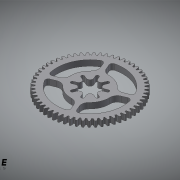
# Autodesk Inventor part: ギアm1z57
Saved by Autodesk Inventor 2020 (Build 240168000, 168)
## iProperties
Part Number: ギアm1z57
Material: 一般
Document SubType Name: Modeling
Designer: Kuroda Akito
Density: 1 g/cm^3
Appearance: 既定
Author: Kuroda Akito
Autodesk Inventor part; units mm, degrees
(part 1 of 3)
ref_plane "YZ Plane" through (0, 0, 0) normal (1, 0, 0) x (0, 1, 0)
ref_plane "XZ Plane" through (0, 0, 0) normal (0, 1, 0) x (-1, 0, 0)
ref_plane "XY Plane" through (0, 0, 0) normal (0, 0, 1) x (1, 0, 0)
sketch "スケッチ1" plane through (0, 0, 0) normal (0, 0, 1) x (1, 0, 0)
  arc A0 (149.035, 132.768) -> (148.9038, 132.247) centre (154.985, 130.9929) ccw
  arc A1 (149.2907, 133.5027) -> (149.035, 132.768) centre (157.2588, 130.3182) ccw
  arc A2 (149.7341, 134.4742) -> (149.2907, 133.5027) centre (159.5839, 129.3913) ccw
  arc A3 (145.977, 132.6583) -> (145.904, 132.1261) centre (152.0862, 131.5485) ccw
  arc A4 (146.1503, 133.4167) -> (145.977, 132.6583) centre (154.4205, 131.128) ccw
  arc A5 (146.4842, 134.431) -> (146.1503, 133.4167) centre (156.8334, 130.4626) ccw
  arc A6 (142.9497, 132.2129) -> (142.9356, 131.6758) centre (149.1439, 131.7819) ccw
  arc A7 (143.0385, 132.9857) -> (142.9497, 132.2129) centre (151.5102, 131.6208) ccw
  arc A8 (143.2588, 134.0307) -> (143.0385, 132.9857) centre (153.9817, 131.2248) ccw
  arc A9 (139.9898, 131.4372) -> (140.0349, 130.9018) centre (146.1937, 131.6901) ccw
  arc A10 (139.993, 132.2151) -> (139.9898, 131.4372) centre (148.5635, 131.7903) ccw
  arc A11 (140.097, 133.2779) -> (139.993, 132.2151) centre (151.0635, 131.6687) ccw
  arc A12 (137.1331, 130.3405) -> (137.2368, 129.8134) centre (143.2716, 131.2744) ccw
  arc A13 (137.0508, 131.1141) -> (137.1331, 130.3405) centre (145.6159, 131.6347) ccw
  arc A14 (137.0372, 132.1819) -> (137.0508, 131.1141) centre (148.1142, 131.7888) ccw
  arc A15 (134.4144, 128.9363) -> (134.5755, 128.4237) centre (140.4129, 130.5398) ccw
  arc A16 (134.2475, 129.6961) -> (134.4144, 128.9363) centre (142.7034, 131.1558) ccw
  arc A17 (134.1165, 130.7559) -> (134.2475, 129.6961) centre (145.1695, 131.5838) ccw
  arc A18 (131.8667, 127.2415) -> (132.0832, 126.7498) centre (137.6524, 129.4952) ccw
  arc A19 (131.6172, 127.9783) -> (131.8667, 127.2415) centre (139.8612, 130.3594) ccw
  arc A20 (131.3705, 129.0173) -> (131.6172, 127.9783) centre (142.2653, 131.0561) ccw
  arc A21 (129.5209, 125.2767) -> (129.7902, 124.8118) centre (135.0236, 128.1532) ccw
  arc A22 (129.1919, 125.9816) -> (129.5209, 125.2767) centre (137.1239, 129.2551) ccw
  arc A23 (128.8323, 126.9871) -> (129.1919, 125.9816) centre (139.4368, 130.2121) ccw
  arc A24 (127.4055, 123.0658) -> (127.7243, 122.6333) centre (132.5583, 126.5301) ccw
  arc A25 (127.0009, 123.7302) -> (127.4055, 123.0658) centre (134.5247, 127.8564) ccw
  arc A26 (126.5329, 124.69) -> (127.0009, 123.7302) centre (136.7182, 129.062) ccw
  arc A27 (125.5462, 120.6355) -> (125.9106, 120.2408) centre (130.2866, 124.6457) ccw
  arc A28 (125.0709, 121.2514) -> (125.5462, 120.6355) centre (132.0951, 126.1803) ccw
  arc A29 (124.5002, 122.154) -> (125.0709, 121.2514) centre (134.1427, 127.6199) ccw
  arc A30 (123.9655, 118.0155) -> (124.3711, 117.6632) centre (128.2359, 122.5229) ccw
  arc A31 (123.4253, 118.5754) -> (123.9655, 118.0155) centre (129.8647, 124.2471) ccw
  arc A32 (122.7588, 119.4097) -> (123.4253, 118.5754) centre (131.7415, 125.9032) ccw
  arc A33 (122.6825, 115.2375) -> (123.1245, 114.932) centre (126.4313, 120.1873) ccw
  arc A34 (122.0841, 115.7346) -> (122.6825, 115.2375) centre (127.8604, 122.0802) ccw
  arc A35 (121.3298, 116.4905) -> (122.0841, 115.7346) centre (129.5437, 123.9327) ccw
  arc A36 (121.713, 112.3353) -> (122.1859, 112.0802) centre (124.8945, 117.6674) ccw
  arc A37 (121.0636, 112.7635) -> (121.713, 112.3353) centre (126.1067, 119.7061) ccw
  arc A38 (120.2307, 113.4318) -> (121.0636, 112.7635) centre (127.576, 121.7325) ccw
  arc A39 (121.0687, 109.344) -> (121.5667, 109.1425) centre (123.6442, 114.9937) ccw
  arc A40 (120.376, 109.6981) -> (121.0687, 109.344) centre (124.6249, 117.1534) ccw
  arc A41 (119.4747, 110.2708) -> (120.376, 109.6981) centre (125.8623, 119.3291) ccw
  arc A42 (120.7573, 106.2999) -> (121.2745, 106.1544) centre (122.6957, 112.1987) ccw
  arc A43 (120.0299, 106.5757) -> (120.7573, 106.2999) centre (123.4328, 114.4531) ccw
  arc A44 (119.071, 107.0458) -> (120.0299, 106.5757) centre (124.4233, 116.7518) ccw
  arc A45 (120.7827, 103.2401) -> (121.3127, 103.1524) centre (122.0604, 109.3163) ccw
  arc A46 (120.0294, 103.4342) -> (120.7827, 103.2401) centre (122.545, 111.6382) ccw
  arc A47 (119.0246, 103.7959) -> (120.0294, 103.4342) centre (123.2767, 114.0318) ccw
  arc A48 (121.1445, 100.2017) -> (121.681, 100.1728) centre (121.746, 106.3816) ccw
  arc A49 (120.3744, 100.3117) -> (121.1445, 100.2017) centre (121.9723, 108.7426) ccw
  arc A50 (119.3359, 100.5607) -> (120.3744, 100.3117) centre (122.4362, 111.2023) ccw
  arc A51 (121.8384, 97.2214) -> (122.3748, 97.2518) centre (121.7564, 103.43) ccw
  arc A52 (121.0608, 97.2461) -> (121.8384, 97.2214) centre (121.7216, 105.8016) ccw
  arc A53 (120.0013, 97.3793) -> (121.0608, 97.2461) centre (121.9121, 108.2974) ccw
  arc A54 (122.8559, 94.3357) -> (123.3857, 94.4248) centre (122.0915, 100.4975) ccw
  arc A55 (122.0804, 94.2747) -> (122.8559, 94.3357) centre (121.7959, 102.8509) ccw
  arc A56 (121.0126, 94.2905) -> (122.0804, 94.2747) centre (121.7107, 105.3525) ccw
  arc A57 (124.1847, 91.5793) -> (124.7015, 91.7262) centre (122.7471, 97.6197) ccw
  arc A58 (123.4206, 91.4334) -> (124.1847, 91.5793) centre (122.1944, 99.9263) ccw
  arc A59 (122.3576, 91.3317) -> (123.4206, 91.4334) centre (121.8345, 102.4033) ccw
  arc A60 (125.8087, 88.9859) -> (126.3062, 89.1887) centre (123.7152, 94.8315) ccw
  arc A61 (125.0653, 88.7568) -> (125.8087, 88.9859) centre (122.9122, 97.0632) ccw
  arc A62 (124.0199, 88.5387) -> (125.0653, 88.7568) centre (122.282, 99.4856) ccw
  arc A63 (127.7081, 86.5869) -> (128.1802, 86.8432) centre (124.9843, 92.1667) ccw
  arc A64 (126.9944, 86.2773) -> (127.7081, 86.5869) centre (123.9406, 94.2966) ccw
  arc A65 (125.9793, 85.9456) -> (126.9944, 86.2773) centre (123.0478, 96.6349) ccw
  arc A66 (129.8599, 84.4113) -> (130.3009, 84.7181) centre (126.5388, 89.6576) ccw
  arc A67 (129.1845, 84.0252) -> (129.8599, 84.4113) centre (125.2672, 91.6598) ccw
  arc A68 (128.2121, 83.5838) -> (129.1845, 84.0252) centre (124.1225, 93.8857) ccw
  arc A69 (132.2379, 82.4857) -> (132.6426, 82.8391) centre (128.3599, 87.3348) ccw
  arc A70 (131.6092, 82.0276) -> (132.2379, 82.4857) centre (126.8757, 89.1849) ccw
  arc A71 (130.6912, 81.482) -> (131.6092, 82.0276) centre (125.4931, 91.2715) ccw
  arc A72 (134.8134, 80.8334) -> (135.1767, 81.2292) centre (130.4254, 85.2265) ccw
  arc A73 (134.2388, 80.3089) -> (134.8134, 80.8334) centre (128.7467, 86.9021) ccw
  arc A74 (133.3865, 79.6656) -> (134.2388, 80.3089) centre (127.143, 88.8238) ccw
  arc A75 (137.555, 79.4744) -> (137.8726, 79.9078) centre (132.7104, 83.3581) ccw
  arc A76 (137.0416, 78.8899) -> (137.555, 79.4744) centre (130.8575, 84.8389) ccw
  arc A77 (136.2652, 78.1567) -> (137.0416, 78.8899) centre (129.0521, 86.5726) ccw
  arc A78 (140.4294, 78.4253) -> (140.6974, 78.891) centre (135.187, 81.7525) ccw
  arc A79 (139.9835, 77.7879) -> (140.4294, 78.4253) centre (133.1825, 83.0204) ccw
  arc A80 (139.2925, 76.9737) -> (139.9835, 77.7879) centre (131.1973, 84.545) ccw
  arc A81 (143.4018, 77.6988) -> (143.617, 78.1911) centre (137.8252, 80.429) ccw
  arc A82 (143.0287, 77.0162) -> (143.4018, 77.6988) centre (135.6934, 81.4688) ccw
  arc A83 (142.4315, 76.1309) -> (143.0287, 77.0162) centre (133.5526, 82.7657) ccw
  arc A84 (146.4361, 77.3036) -> (146.5958, 77.8166) centre (140.593, 79.4039) ccw
  arc A85 (146.1404, 76.5841) -> (146.4361, 77.3036) centre (138.3598, 80.2028) ccw
  arc A86 (145.6441, 75.6386) -> (146.1404, 76.5841) centre (136.0892, 81.2563) ccw
  arc A87 (149.4955, 77.2447) -> (149.5978, 77.7721) centre (143.4568, 78.6894) ccw
  arc A88 (149.2807, 76.497) -> (149.4955, 77.2447) centre (141.1492, 79.2378) ccw
  arc A89 (148.8915, 75.5026) -> (149.2807, 76.497) centre (138.7766, 80.0351) ccw
  arc A90 (152.5428, 77.5227) -> (152.5864, 78.0581) centre (146.3818, 78.2943) ccw
  arc A91 (152.4115, 76.7559) -> (152.5428, 77.5227) centre (144.0279, 78.5855) ccw
  arc A92 (152.134, 75.7247) -> (152.4115, 76.7559) centre (141.5819, 79.117) ccw
  arc A93 (155.541, 78.1342) -> (155.5254, 78.6712) centre (149.3325, 78.2233) ccw
  arc A94 (155.4949, 77.3576) -> (155.541, 78.1342) centre (146.9608, 78.2538) ccw
  arc A95 (155.3325, 76.3021) -> (155.4949, 77.3576) centre (144.4713, 78.513) ccw
  arc A96 (158.4537, 79.0718) -> (158.3792, 79.6038) centre (152.2731, 78.4774) ccw
  arc A97 (158.4933, 78.2949) -> (158.4537, 79.0718) centre (149.9125, 78.2468) ccw
  arc A98 (158.448, 77.228) -> (158.4933, 78.2949) centre (147.4095, 78.2306) ccw
  arc A99 (161.2456, 80.3241) -> (161.113, 80.8448) centre (155.1679, 79.0535) ccw
  arc A100 (161.3704, 79.5563) -> (161.2456, 80.3241) centre (152.847, 78.5646) ccw
  arc A101 (161.4428, 78.4909) -> (161.3704, 79.5563) centre (150.361, 78.2731) ccw
  arc A102 (163.8828, 81.876) -> (163.6937, 82.3789) centre (157.9817, 79.9445) ccw
  arc A103 (164.0913, 81.1266) -> (163.8828, 81.876) centre (155.7287, 79.2032) ccw
  arc A104 (164.2805, 80.0756) -> (164.0913, 81.1266) centre (153.2899, 78.64) ccw
  arc A105 (166.3332, 83.7086) -> (166.09, 84.1876) centre (160.6805, 81.1396) ccw
  arc A106 (166.623, 82.9867) -> (166.3332, 83.7086) centre (158.5227, 80.155) ccw
  arc A107 (166.9266, 81.9628) -> (166.623, 82.9867) centre (156.1606, 79.3269) ccw
  arc A108 (168.5672, 85.7996) -> (168.2728, 86.249) centre (163.2314, 82.6244) ccw
  arc A109 (168.9346, 85.1139) -> (168.5672, 85.7996) centre (161.195, 81.4084) ccw
  arc A110 (169.349, 84.1297) -> (168.9346, 85.1139) centre (158.9383, 80.3255) ccw
  arc A111 (170.5576, 88.1237) -> (170.2155, 88.538) centre (165.6035, 84.3808) ccw
  arc A112 (170.9982, 87.4826) -> (170.5576, 88.1237) centre (163.7132, 82.9481) ccw
  arc A113 (171.5184, 86.55) -> (170.9982, 87.4826) centre (161.5894, 81.6236) ccw
  arc A114 (172.2803, 90.6527) -> (171.8947, 91.0268) centre (167.768, 86.3874) ccw
  arc A115 (172.7887, 90.0639) -> (172.2803, 90.6527) centre (166.0468, 84.7555) ccw
  arc A116 (173.4083, 89.1942) -> (172.7887, 90.0639) centre (164.0815, 83.2054) ccw
  arc A117 (173.7143, 93.3558) -> (173.2899, 93.6852) centre (169.6986, 88.62) ccw
  arc A118 (174.2844, 92.8265) -> (173.7143, 93.3558) centre (168.1673, 86.8087) ccw
  arc A119 (174.9959, 92.0302) -> (174.2844, 92.8265) centre (166.3846, 85.0518) ccw
  arc A120 (174.8422, 96.2002) -> (174.3841, 96.481) centre (171.3719, 91.0515) ccw
  arc A121 (175.4671, 95.7369) -> (174.8422, 96.2002) centre (170.0491, 89.0827) ccw
  arc A122 (176.2619, 95.0237) -> (175.4671, 95.7369) centre (168.4705, 87.1403) ccw
  arc A123 (175.6504, 99.1515) -> (175.1642, 99.3801) centre (172.7675, 93.6522) ccw
  arc A124 (176.3224, 98.7597) -> (175.6504, 99.1515) centre (171.6694, 91.5499) ccw
  arc A125 (177.1909, 98.1383) -> (176.3224, 98.7597) centre (170.314, 89.4456) ccw
  arc A126 (176.129, 102.1738) -> (175.6206, 102.3475) centre (173.8685, 96.3907) ccw
  arc A127 (176.8401, 101.8583) -> (176.129, 102.1738) centre (173.0084, 94.1803) ccw
  arc A128 (177.7716, 101.3362) -> (176.8401, 101.8583) centre (171.8927, 91.9397) ccw
  arc A129 (176.2722, 105.2303) -> (175.7478, 105.3471) centre (174.6617, 99.2337) ccw
  arc A130 (177.0137, 104.995) -> (176.2722, 105.2303) centre (174.0499, 96.9421) ccw
  arc A131 (177.997, 104.5785) -> (177.0137, 104.995) centre (173.1875, 94.5924) ccw
  arc A132 (176.0783, 108.2841) -> (175.5442, 108.3425) centre (175.1372, 102.1467) ccw
  arc A133 (176.8412, 108.1318) -> (176.0783, 108.2841) centre (174.7813, 99.8017) ccw
  arc A134 (177.8643, 107.826) -> (176.8412, 108.1318) centre (174.1826, 97.3714) ccw
  arc A135 (175.5496, 111.298) -> (175.0124, 111.2973) centre (175.2894, 105.0943) ccw
  arc A136 (176.3246, 111.2305) -> (175.5496, 111.298) centre (175.1936, 102.7244) ccw
  arc A137 (177.3752, 111.0392) -> (176.3246, 111.2305) centre (174.8659, 100.243) ccw
  arc A138 (174.6926, 114.2355) -> (174.1587, 114.1756) centre (175.1165, 108.0408) ccw
  arc A139 (175.4703, 114.2537) -> (174.6926, 114.2355) centre (175.2819, 105.6748) ccw
  arc A140 (176.5356, 114.179) -> (175.4703, 114.2537) centre (175.2292, 103.1723) ccw
  arc A141 (173.5177, 117.0608) -> (172.9936, 116.9426) centre (174.6204, 110.9504) ccw
  arc A142 (174.2887, 117.1645) -> (173.5177, 117.0608) centre (175.0451, 108.6169) ccw
  arc A143 (175.3557, 117.2075) -> (174.2887, 117.1645) centre (175.268, 106.1238) ccw
  arc A144 (172.0391, 119.7398) -> (171.5312, 119.5646) centre (173.8073, 113.7878) ccw
  arc A145 (172.794, 119.9276) -> (172.0391, 119.7398) centre (174.4861, 111.5151) ccw
  arc A146 (173.8498, 120.0877) -> (172.794, 119.9276) centre (174.9819, 109.0617) ccw
  arc A147 (170.2747, 122.2398) -> (169.7891, 122.0099) centre (172.687, 116.5184) ccw
  arc A148 (171.0044, 122.5095) -> (170.2747, 122.2398) centre (173.6117, 114.3343) ccw
  arc A149 (172.0361, 122.7848) -> (171.0044, 122.5095) centre (174.3744, 111.9503) ccw
  arc A150 (168.246, 124.5306) -> (167.7887, 124.2486) centre (171.273, 119.1093) ccw
  arc A151 (168.9416, 124.8789) -> (168.246, 124.5306) centre (172.4325, 117.0401) ccw
  arc A152 (169.9368, 125.2661) -> (168.9416, 124.8789) centre (173.4528, 114.7545) ccw
  arc A153 (165.9777, 126.5843) -> (165.5541, 126.2537) centre (169.5827, 121.5289) ccw
  arc A154 (166.6307, 127.007) -> (165.9777, 126.5843) centre (170.9627, 119.5998) ccw
  arc A155 (167.5773, 127.5013) -> (166.6307, 127.007) centre (172.2282, 117.4403) ccw
  arc A156 (163.4971, 128.3759) -> (163.1125, 128.0008) centre (167.6364, 123.7478) ccw
  arc A157 (164.0997, 128.868) -> (163.4971, 128.3759) centre (169.2203, 121.9823) ccw
  arc A158 (164.9862, 129.4634) -> (164.0997, 128.868) centre (170.7157, 119.9751) ccw
  arc A159 (160.8346, 129.8839) -> (160.4936, 129.4687) centre (165.4579, 125.7392) ccw
  arc A160 (161.3793, 130.4392) -> (160.8346, 129.8839) centre (167.2263, 124.1586) ccw
  arc A161 (162.1949, 131.1285) -> (161.3793, 130.4392) centre (168.9335, 122.3281) ccw
  arc A162 (158.0223, 131.0897) -> (157.729, 130.6396) centre (163.0734, 127.4788) ccw
  arc A163 (158.5026, 131.7016) -> (158.0223, 131.0897) centre (165.005, 126.1024) ccw
  arc A164 (159.2375, 132.4765) -> (158.5026, 131.7016) centre (166.9032, 124.4708) ccw
  arc A165 (155.0944, 131.9789) -> (154.8525, 131.4992) centre (160.5121, 128.9456) ccw
  arc A166 (155.5045, 132.6399) -> (155.0944, 131.9789) centre (162.5834, 127.79) ccw
  arc A167 (156.1497, 133.4909) -> (155.5045, 132.6399) centre (164.6496, 126.3771) ccw
  arc A168 (152.0865, 132.5406) -> (151.8988, 132.0372) centre (157.805, 130.1217) ccw
  arc A169 (152.4214, 133.2427) -> (152.0865, 132.5406) centre (159.9909, 129.201) ccw
  arc A170 (152.969, 134.1595) -> (152.4214, 133.2427) centre (162.1999, 128.024) ccw
  arc A171 (148.0962, 132.247) -> (147.965, 132.768) centre (142.015, 130.9929) ccw
  arc A172 (147.965, 132.768) -> (147.7093, 133.5027) centre (139.7412, 130.3182) ccw
  arc A173 (147.7093, 133.5027) -> (147.2659, 134.4742) centre (137.4161, 129.3913) ccw
  arc A174 (145.1012, 132.0372) -> (144.9135, 132.5406) centre (139.195, 130.1217) ccw
  arc A175 (144.9135, 132.5406) -> (144.5786, 133.2427) centre (137.0091, 129.201) ccw
  arc A176 (144.5786, 133.2427) -> (144.031, 134.1595) centre (134.8001, 128.024) ccw
  arc A177 (142.1475, 131.4992) -> (141.9056, 131.9789) centre (136.4879, 128.9456) ccw
  arc A178 (141.9056, 131.9789) -> (141.4955, 132.6399) centre (134.4166, 127.79) ccw
  arc A179 (141.4955, 132.6399) -> (140.8503, 133.4909) centre (132.3504, 126.3771) ccw
  arc A180 (139.271, 130.6396) -> (138.9777, 131.0897) centre (133.9266, 127.4788) ccw
  arc A181 (138.9777, 131.0897) -> (138.4974, 131.7016) centre (131.995, 126.1024) ccw
  arc A182 (138.4974, 131.7016) -> (137.7625, 132.4765) centre (130.0968, 124.4708) ccw
  arc A183 (136.5064, 129.4687) -> (136.1654, 129.8839) centre (131.5421, 125.7392) ccw
  arc A184 (136.1654, 129.8839) -> (135.6207, 130.4392) centre (129.7737, 124.1586) ccw
  arc A185 (135.6207, 130.4392) -> (134.8051, 131.1285) centre (128.0665, 122.3281) ccw
  arc A186 (133.8875, 128.0008) -> (133.5029, 128.3759) centre (129.3636, 123.7478) ccw
  arc A187 (133.5029, 128.3759) -> (132.9003, 128.868) centre (127.7797, 121.9823) ccw
  arc A188 (132.9003, 128.868) -> (132.0138, 129.4634) centre (126.2843, 119.9751) ccw
  arc A189 (131.4459, 126.2537) -> (131.0223, 126.5843) centre (127.4173, 121.5289) ccw
  arc A190 (131.0223, 126.5843) -> (130.3693, 127.007) centre (126.0373, 119.5998) ccw
  arc A191 (130.3693, 127.007) -> (129.4227, 127.5013) centre (124.7718, 117.4403) ccw
  arc A192 (129.2113, 124.2486) -> (128.754, 124.5306) centre (125.727, 119.1093) ccw
  arc A193 (128.754, 124.5306) -> (128.0584, 124.8789) centre (124.5675, 117.0401) ccw
  arc A194 (128.0584, 124.8789) -> (127.0632, 125.2661) centre (123.5472, 114.7545) ccw
  arc A195 (127.2109, 122.0099) -> (126.7253, 122.2398) centre (124.313, 116.5184) ccw
  arc A196 (126.7253, 122.2398) -> (125.9956, 122.5095) centre (123.3883, 114.3343) ccw
  arc A197 (125.9956, 122.5095) -> (124.9639, 122.7848) centre (122.6256, 111.9503) ccw
  arc A198 (125.4688, 119.5646) -> (124.9609, 119.7398) centre (123.1927, 113.7878) ccw
  arc A199 (124.9609, 119.7398) -> (124.206, 119.9276) centre (122.5139, 111.5151) ccw
  arc A200 (124.206, 119.9276) -> (123.1502, 120.0877) centre (122.0181, 109.0617) ccw
  arc A201 (124.0064, 116.9426) -> (123.4823, 117.0608) centre (122.3796, 110.9504) ccw
  arc A202 (123.4823, 117.0608) -> (122.7113, 117.1645) centre (121.9549, 108.6169) ccw
  arc A203 (122.7113, 117.1645) -> (121.6443, 117.2075) centre (121.732, 106.1238) ccw
  arc A204 (122.8413, 114.1756) -> (122.3074, 114.2355) centre (121.8835, 108.0408) ccw
  arc A205 (122.3074, 114.2355) -> (121.5297, 114.2537) centre (121.7181, 105.6748) ccw
  arc A206 (121.5297, 114.2537) -> (120.4644, 114.179) centre (121.7708, 103.1723) ccw
  arc A207 (121.9876, 111.2973) -> (121.4504, 111.298) centre (121.7106, 105.0943) ccw
  arc A208 (121.4504, 111.298) -> (120.6754, 111.2305) centre (121.8064, 102.7244) ccw
  arc A209 (120.6754, 111.2305) -> (119.6248, 111.0392) centre (122.1341, 100.243) ccw
  arc A210 (121.4558, 108.3425) -> (120.9217, 108.2841) centre (121.8628, 102.1467) ccw
  arc A211 (120.9217, 108.2841) -> (120.1588, 108.1318) centre (122.2187, 99.8017) ccw
  arc A212 (120.1588, 108.1318) -> (119.1357, 107.826) centre (122.8174, 97.3714) ccw
  arc A213 (121.2522, 105.3471) -> (120.7278, 105.2303) centre (122.3383, 99.2337) ccw
  arc A214 (120.7278, 105.2303) -> (119.9863, 104.995) centre (122.9501, 96.9421) ccw
  arc A215 (119.9863, 104.995) -> (119.003, 104.5785) centre (123.8125, 94.5924) ccw
  arc A216 (121.3794, 102.3475) -> (120.871, 102.1738) centre (123.1315, 96.3907) ccw
  arc A217 (120.871, 102.1738) -> (120.1599, 101.8583) centre (123.9916, 94.1803) ccw
  arc A218 (120.1599, 101.8583) -> (119.2284, 101.3362) centre (125.1073, 91.9397) ccw
  arc A219 (121.8358, 99.3801) -> (121.3496, 99.1515) centre (124.2325, 93.6522) ccw
  arc A220 (121.3496, 99.1515) -> (120.6776, 98.7597) centre (125.3306, 91.5499) ccw
  arc A221 (120.6776, 98.7597) -> (119.8091, 98.1383) centre (126.686, 89.4456) ccw
  arc A222 (122.6159, 96.481) -> (122.1578, 96.2002) centre (125.6281, 91.0515) ccw
  arc A223 (122.1578, 96.2002) -> (121.5329, 95.7369) centre (126.9509, 89.0827) ccw
  arc A224 (121.5329, 95.7369) -> (120.7381, 95.0237) centre (128.5295, 87.1403) ccw
  arc A225 (123.7101, 93.6852) -> (123.2857, 93.3558) centre (127.3014, 88.62) ccw
  arc A226 (123.2857, 93.3558) -> (122.7156, 92.8265) centre (128.8327, 86.8087) ccw
  arc A227 (122.7156, 92.8265) -> (122.0041, 92.0302) centre (130.6154, 85.0518) ccw
  arc A228 (125.1053, 91.0268) -> (124.7197, 90.6527) centre (129.232, 86.3874) ccw
  arc A229 (124.7197, 90.6527) -> (124.2113, 90.0639) centre (130.9532, 84.7555) ccw
  arc A230 (124.2113, 90.0639) -> (123.5917, 89.1942) centre (132.9185, 83.2054) ccw
  arc A231 (126.7845, 88.538) -> (126.4424, 88.1237) centre (131.3965, 84.3808) ccw
  arc A232 (126.4424, 88.1237) -> (126.0018, 87.4826) centre (133.2868, 82.9481) ccw
  arc A233 (126.0018, 87.4826) -> (125.4816, 86.55) centre (135.4106, 81.6236) ccw
  arc A234 (128.7272, 86.249) -> (128.4328, 85.7996) centre (133.7686, 82.6244) ccw
  arc A235 (128.4328, 85.7996) -> (128.0654, 85.1139) centre (135.805, 81.4084) ccw
  arc A236 (128.0654, 85.1139) -> (127.651, 84.1297) centre (138.0617, 80.3255) ccw
  arc A237 (130.91, 84.1876) -> (130.6668, 83.7086) centre (136.3195, 81.1396) ccw
  arc A238 (130.6668, 83.7086) -> (130.377, 82.9867) centre (138.4773, 80.155) ccw
  arc A239 (130.377, 82.9867) -> (130.0734, 81.9628) centre (140.8394, 79.3269) ccw
  arc A240 (133.3063, 82.3789) -> (133.1172, 81.876) centre (139.0183, 79.9445) ccw
  arc A241 (133.1172, 81.876) -> (132.9087, 81.1266) centre (141.2713, 79.2032) ccw
  arc A242 (132.9087, 81.1266) -> (132.7195, 80.0756) centre (143.7101, 78.64) ccw
  arc A243 (135.887, 80.8448) -> (135.7544, 80.3241) centre (141.8321, 79.0535) ccw
  arc A244 (135.7544, 80.3241) -> (135.6296, 79.5563) centre (144.153, 78.5646) ccw
  arc A245 (135.6296, 79.5563) -> (135.5572, 78.4909) centre (146.639, 78.2731) ccw
  arc A246 (138.6208, 79.6038) -> (138.5463, 79.0718) centre (144.7269, 78.4774) ccw
  arc A247 (138.5463, 79.0718) -> (138.5067, 78.2949) centre (147.0875, 78.2468) ccw
  arc A248 (138.5067, 78.2949) -> (138.552, 77.228) centre (149.5905, 78.2306) ccw
  arc A249 (141.4746, 78.6712) -> (141.459, 78.1342) centre (147.6675, 78.2233) ccw
  arc A250 (141.459, 78.1342) -> (141.5051, 77.3576) centre (150.0392, 78.2538) ccw
  arc A251 (141.5051, 77.3576) -> (141.6675, 76.3021) centre (152.5287, 78.513) ccw
  arc A252 (144.4136, 78.0581) -> (144.4572, 77.5227) centre (150.6182, 78.2943) ccw
  arc A253 (144.4572, 77.5227) -> (144.5885, 76.7559) centre (152.9721, 78.5855) ccw
  arc A254 (144.5885, 76.7559) -> (144.866, 75.7247) centre (155.4181, 79.117) ccw
  arc A255 (147.4022, 77.7721) -> (147.5045, 77.2447) centre (153.5432, 78.6894) ccw
  arc A256 (147.5045, 77.2447) -> (147.7193, 76.497) centre (155.8508, 79.2378) ccw
  arc A257 (147.7193, 76.497) -> (148.1085, 75.5026) centre (158.2234, 80.0351) ccw
  arc A258 (150.4042, 77.8166) -> (150.5639, 77.3036) centre (156.407, 79.4039) ccw
  arc A259 (150.5639, 77.3036) -> (150.8596, 76.5841) centre (158.6402, 80.2028) ccw
  arc A260 (150.8596, 76.5841) -> (151.3559, 75.6386) centre (160.9108, 81.2563) ccw
  arc A261 (153.383, 78.1911) -> (153.5982, 77.6988) centre (159.1748, 80.429) ccw
  arc A262 (153.5982, 77.6988) -> (153.9713, 77.0162) centre (161.3066, 81.4688) ccw
  arc A263 (153.9713, 77.0162) -> (154.5685, 76.1309) centre (163.4474, 82.7657) ccw
  arc A264 (156.3026, 78.891) -> (156.5706, 78.4253) centre (161.813, 81.7525) ccw
  arc A265 (156.5706, 78.4253) -> (157.0165, 77.7879) centre (163.8175, 83.0204) ccw
  arc A266 (157.0165, 77.7879) -> (157.7075, 76.9737) centre (165.8027, 84.545) ccw
  arc A267 (159.1274, 79.9078) -> (159.445, 79.4744) centre (164.2896, 83.3581) ccw
  arc A268 (159.445, 79.4744) -> (159.9584, 78.8899) centre (166.1425, 84.8389) ccw
  arc A269 (159.9584, 78.8899) -> (160.7348, 78.1567) centre (167.9479, 86.5726) ccw
  arc A270 (161.8233, 81.2292) -> (162.1866, 80.8334) centre (166.5746, 85.2265) ccw
  arc A271 (162.1866, 80.8334) -> (162.7612, 80.3089) centre (168.2533, 86.9021) ccw
  arc A272 (162.7612, 80.3089) -> (163.6135, 79.6656) centre (169.857, 88.8238) ccw
  arc A273 (164.3574, 82.8391) -> (164.7621, 82.4857) centre (168.6401, 87.3348) ccw
  arc A274 (164.7621, 82.4857) -> (165.3908, 82.0276) centre (170.1243, 89.1849) ccw
  arc A275 (165.3908, 82.0276) -> (166.3088, 81.482) centre (171.5069, 91.2715) ccw
  arc A276 (166.6991, 84.7181) -> (167.1401, 84.4113) centre (170.4612, 89.6576) ccw
  arc A277 (167.1401, 84.4113) -> (167.8155, 84.0252) centre (171.7328, 91.6598) ccw
  arc A278 (167.8155, 84.0252) -> (168.7879, 83.5838) centre (172.8775, 93.8857) ccw
  arc A279 (168.8198, 86.8432) -> (169.2919, 86.5869) centre (172.0157, 92.1667) ccw
  arc A280 (169.2919, 86.5869) -> (170.0056, 86.2773) centre (173.0594, 94.2966) ccw
  arc A281 (170.0056, 86.2773) -> (171.0207, 85.9456) centre (173.9522, 96.6349) ccw
  arc A282 (170.6938, 89.1887) -> (171.1913, 88.9859) centre (173.2848, 94.8315) ccw
  arc A283 (171.1913, 88.9859) -> (171.9347, 88.7568) centre (174.0878, 97.0632) ccw
  arc A284 (171.9347, 88.7568) -> (172.9801, 88.5387) centre (174.718, 99.4856) ccw
  arc A285 (172.2985, 91.7262) -> (172.8153, 91.5793) centre (174.2529, 97.6197) ccw
  arc A286 (172.8153, 91.5793) -> (173.5794, 91.4334) centre (174.8056, 99.9263) ccw
  arc A287 (173.5794, 91.4334) -> (174.6424, 91.3317) centre (175.1655, 102.4033) ccw
  arc A288 (173.6143, 94.4248) -> (174.1441, 94.3357) centre (174.9085, 100.4975) ccw
  arc A289 (174.1441, 94.3357) -> (174.9196, 94.2747) centre (175.2041, 102.8509) ccw
  arc A290 (174.9196, 94.2747) -> (175.9874, 94.2905) centre (175.2893, 105.3525) ccw
  arc A291 (174.6252, 97.2518) -> (175.1616, 97.2214) centre (175.2436, 103.43) ccw
  arc A292 (175.1616, 97.2214) -> (175.9392, 97.2461) centre (175.2784, 105.8016) ccw
  arc A293 (175.9392, 97.2461) -> (176.9987, 97.3793) centre (175.0879, 108.2974) ccw
  arc A294 (175.319, 100.1728) -> (175.8555, 100.2017) centre (175.254, 106.3816) ccw
  arc A295 (175.8555, 100.2017) -> (176.6256, 100.3117) centre (175.0277, 108.7426) ccw
  arc A296 (176.6256, 100.3117) -> (177.6641, 100.5607) centre (174.5638, 111.2023) ccw
  arc A297 (175.6873, 103.1524) -> (176.2173, 103.2401) centre (174.9396, 109.3163) ccw
  arc A298 (176.2173, 103.2401) -> (176.9706, 103.4342) centre (174.455, 111.6382) ccw
  arc A299 (176.9706, 103.4342) -> (177.9754, 103.7959) centre (173.7233, 114.0318) ccw
  arc A300 (175.7255, 106.1544) -> (176.2427, 106.2999) centre (174.3043, 112.1987) ccw
  arc A301 (176.2427, 106.2999) -> (176.9701, 106.5757) centre (173.5672, 114.4531) ccw
  arc A302 (176.9701, 106.5757) -> (177.929, 107.0458) centre (172.5767, 116.7518) ccw
  arc A303 (175.4333, 109.1425) -> (175.9313, 109.344) centre (173.3558, 114.9937) ccw
  arc A304 (175.9313, 109.344) -> (176.624, 109.6981) centre (172.3751, 117.1534) ccw
  arc A305 (176.624, 109.6981) -> (177.5253, 110.2708) centre (171.1377, 119.3291) ccw
  arc A306 (174.8141, 112.0802) -> (175.287, 112.3353) centre (172.1055, 117.6674) ccw
  arc A307 (175.287, 112.3353) -> (175.9364, 112.7635) centre (170.8933, 119.7061) ccw
  arc A308 (175.9364, 112.7635) -> (176.7693, 113.4318) centre (169.424, 121.7325) ccw
  arc A309 (173.8755, 114.932) -> (174.3175, 115.2375) centre (170.5687, 120.1873) ccw
  arc A310 (174.3175, 115.2375) -> (174.9159, 115.7346) centre (169.1396, 122.0802) ccw
  arc A311 (174.9159, 115.7346) -> (175.6702, 116.4905) centre (167.4563, 123.9327) ccw
  arc A312 (172.6289, 117.6632) -> (173.0345, 118.0155) centre (168.7641, 122.5229) ccw
  arc A313 (173.0345, 118.0155) -> (173.5747, 118.5754) centre (167.1353, 124.2471) ccw
  arc A314 (173.5747, 118.5754) -> (174.2412, 119.4097) centre (165.2585, 125.9032) ccw
  arc A315 (171.0894, 120.2408) -> (171.4538, 120.6355) centre (166.7134, 124.6457) ccw
  arc A316 (171.4538, 120.6355) -> (171.9291, 121.2514) centre (164.9049, 126.1803) ccw
  arc A317 (171.9291, 121.2514) -> (172.4998, 122.154) centre (162.8573, 127.6199) ccw
  arc A318 (169.2757, 122.6333) -> (169.5945, 123.0658) centre (164.4417, 126.5301) ccw
  arc A319 (169.5945, 123.0658) -> (169.9991, 123.7302) centre (162.4753, 127.8564) ccw
  arc A320 (169.9991, 123.7302) -> (170.4671, 124.69) centre (160.2818, 129.062) ccw
  arc A321 (167.2098, 124.8118) -> (167.4791, 125.2767) centre (161.9764, 128.1532) ccw
  arc A322 (167.4791, 125.2767) -> (167.8081, 125.9816) centre (159.8761, 129.2551) ccw
  arc A323 (167.8081, 125.9816) -> (168.1677, 126.9871) centre (157.5632, 130.2121) ccw
  arc A324 (164.9168, 126.7498) -> (165.1333, 127.2415) centre (159.3476, 129.4952) ccw
  arc A325 (165.1333, 127.2415) -> (165.3828, 127.9783) centre (157.1388, 130.3594) ccw
  arc A326 (165.3828, 127.9783) -> (165.6295, 129.0173) centre (154.7347, 131.0561) ccw
  arc A327 (162.4245, 128.4237) -> (162.5856, 128.9363) centre (156.5871, 130.5398) ccw
  arc A328 (162.5856, 128.9363) -> (162.7525, 129.6961) centre (154.2966, 131.1558) ccw
  arc A329 (162.7525, 129.6961) -> (162.8835, 130.7559) centre (151.8305, 131.5838) ccw
  arc A330 (159.7632, 129.8134) -> (159.8669, 130.3405) centre (153.7284, 131.2744) ccw
  arc A331 (159.8669, 130.3405) -> (159.9492, 131.1141) centre (151.3841, 131.6347) ccw
  arc A332 (159.9492, 131.1141) -> (159.9628, 132.1819) centre (148.8858, 131.7888) ccw
  arc A333 (156.9651, 130.9018) -> (157.0102, 131.4372) centre (150.8063, 131.6901) ccw
  arc A334 (157.0102, 131.4372) -> (157.007, 132.2151) centre (148.4365, 131.7903) ccw
  arc A335 (157.007, 132.2151) -> (156.903, 133.2779) centre (145.9365, 131.6687) ccw
  arc A336 (154.0644, 131.6758) -> (154.0503, 132.2129) centre (147.8561, 131.7819) ccw
  arc A337 (154.0503, 132.2129) -> (153.9615, 132.9857) centre (145.4898, 131.6208) ccw
  arc A338 (153.9615, 132.9857) -> (153.7412, 134.0307) centre (143.0183, 131.2248) ccw
  arc A339 (151.096, 132.1261) -> (151.023, 132.6583) centre (144.9138, 131.5485) ccw
  arc A340 (151.023, 132.6583) -> (150.8497, 133.4167) centre (142.5795, 131.128) ccw
  arc A341 (150.8497, 133.4167) -> (150.5158, 134.431) centre (140.1666, 130.4626) ccw
  arc A342 (148.9038, 132.247) -> (148.0962, 132.247) centre (148.5, 105) ccw
  arc A343 (145.904, 132.1261) -> (145.1012, 132.0372) centre (148.5, 105) ccw
  arc A344 (142.9356, 131.6758) -> (142.1475, 131.4992) centre (148.5, 105) ccw
  arc A345 (140.0349, 130.9018) -> (139.271, 130.6396) centre (148.5, 105) ccw
  arc A346 (137.2368, 129.8134) -> (136.5064, 129.4687) centre (148.5, 105) ccw
  arc A347 (134.5755, 128.4237) -> (133.8875, 128.0008) centre (148.5, 105) ccw
  arc A348 (132.0832, 126.7498) -> (131.4459, 126.2537) centre (148.5, 105) ccw
  arc A349 (129.7902, 124.8118) -> (129.2113, 124.2486) centre (148.5, 105) ccw
  arc A350 (127.7243, 122.6333) -> (127.2109, 122.0099) centre (148.5, 105) ccw
  arc A351 (125.9106, 120.2408) -> (125.4688, 119.5646) centre (148.5, 105) ccw
  arc A352 (124.3711, 117.6632) -> (124.0064, 116.9426) centre (148.5, 105) ccw
  arc A353 (123.1245, 114.932) -> (122.8413, 114.1756) centre (148.5, 105) ccw
  arc A354 (122.1859, 112.0802) -> (121.9876, 111.2973) centre (148.5, 105) ccw
  arc A355 (121.5667, 109.1425) -> (121.4558, 108.3425) centre (148.5, 105) ccw
  arc A356 (121.2745, 106.1544) -> (121.2522, 105.3471) centre (148.5, 105) ccw
  arc A357 (121.3127, 103.1524) -> (121.3794, 102.3475) centre (148.5, 105) ccw
  arc A358 (121.681, 100.1728) -> (121.8358, 99.3801) centre (148.5, 105) ccw
  arc A359 (122.3748, 97.2518) -> (122.6159, 96.481) centre (148.5, 105) ccw
  arc A360 (123.3857, 94.4248) -> (123.7101, 93.6852) centre (148.5, 105) ccw
  arc A361 (124.7015, 91.7262) -> (125.1053, 91.0268) centre (148.5, 105) ccw
  arc A362 (126.3062, 89.1887) -> (126.7845, 88.538) centre (148.5, 105) ccw
  arc A363 (128.1802, 86.8432) -> (128.7272, 86.249) centre (148.5, 105) ccw
  arc A364 (130.3009, 84.7181) -> (130.91, 84.1876) centre (148.5, 105) ccw
  arc A365 (132.6426, 82.8391) -> (133.3063, 82.3789) centre (148.5, 105) ccw
  arc A366 (135.1767, 81.2292) -> (135.887, 80.8448) centre (148.5, 105) ccw
  arc A367 (137.8726, 79.9078) -> (138.6208, 79.6038) centre (148.5, 105) ccw
  arc A368 (140.6974, 78.891) -> (141.4746, 78.6712) centre (148.5, 105) ccw
  arc A369 (143.617, 78.1911) -> (144.4136, 78.0581) centre (148.5, 105) ccw
  arc A370 (146.5958, 77.8166) -> (147.4022, 77.7721) centre (148.5, 105) ccw
  arc A371 (149.5978, 77.7721) -> (150.4042, 77.8166) centre (148.5, 105) ccw
  arc A372 (152.5864, 78.0581) -> (153.383, 78.1911) centre (148.5, 105) ccw
  arc A373 (155.5254, 78.6712) -> (156.3026, 78.891) centre (148.5, 105) ccw
  arc A374 (158.3792, 79.6038) -> (159.1274, 79.9078) centre (148.5, 105) ccw
  arc A375 (161.113, 80.8448) -> (161.8233, 81.2292) centre (148.5, 105) ccw
  arc A376 (163.6937, 82.3789) -> (164.3574, 82.8391) centre (148.5, 105) ccw
  arc A377 (166.09, 84.1876) -> (166.6991, 84.7181) centre (148.5, 105) ccw
  arc A378 (168.2728, 86.249) -> (168.8198, 86.8432) centre (148.5, 105) ccw
  arc A379 (170.2155, 88.538) -> (170.6938, 89.1887) centre (148.5, 105) ccw
  arc A380 (171.8947, 91.0268) -> (172.2985, 91.7262) centre (148.5, 105) ccw
  arc A381 (173.2899, 93.6852) -> (173.6143, 94.4248) centre (148.5, 105) ccw
  arc A382 (174.3841, 96.481) -> (174.6252, 97.2518) centre (148.5, 105) ccw
  arc A383 (175.1642, 99.3801) -> (175.319, 100.1728) centre (148.5, 105) ccw
  arc A384 (175.6206, 102.3475) -> (175.6873, 103.1524) centre (148.5, 105) ccw
  arc A385 (175.7478, 105.3471) -> (175.7255, 106.1544) centre (148.5, 105) ccw
  arc A386 (175.5442, 108.3425) -> (175.4333, 109.1425) centre (148.5, 105) ccw
  arc A387 (175.0124, 111.2973) -> (174.8141, 112.0802) centre (148.5, 105) ccw
  arc A388 (174.1587, 114.1756) -> (173.8755, 114.932) centre (148.5, 105) ccw
  arc A389 (172.9936, 116.9426) -> (172.6289, 117.6632) centre (148.5, 105) ccw
  arc A390 (171.5312, 119.5646) -> (171.0894, 120.2408) centre (148.5, 105) ccw
  arc A391 (169.7891, 122.0099) -> (169.2757, 122.6333) centre (148.5, 105) ccw
  arc A392 (167.7887, 124.2486) -> (167.2098, 124.8118) centre (148.5, 105) ccw
  arc A393 (165.5541, 126.2537) -> (164.9168, 126.7498) centre (148.5, 105) ccw
  arc A394 (163.1125, 128.0008) -> (162.4245, 128.4237) centre (148.5, 105) ccw
  arc A395 (160.4936, 129.4687) -> (159.7632, 129.8134) centre (148.5, 105) ccw
  arc A396 (157.729, 130.6396) -> (156.9651, 130.9018) centre (148.5, 105) ccw
  arc A397 (154.8525, 131.4992) -> (154.0644, 131.6758) centre (148.5, 105) ccw
  arc A398 (151.8988, 132.0372) -> (151.096, 132.1261) centre (148.5, 105) ccw
  arc A399 (147.2659, 134.4742) -> (146.4842, 134.431) centre (148.5, 105) ccw
  arc A400 (144.031, 134.1595) -> (143.2588, 134.0307) centre (148.5, 105) ccw
  arc A401 (140.8503, 133.4909) -> (140.097, 133.2779) centre (148.5, 105) ccw
  arc A402 (137.7625, 132.4765) -> (137.0372, 132.1819) centre (148.5, 105) ccw
  arc A403 (134.8051, 131.1285) -> (134.1165, 130.7559) centre (148.5, 105) ccw
  arc A404 (132.0138, 129.4634) -> (131.3705, 129.0173) centre (148.5, 105) ccw
  arc A405 (129.4227, 127.5013) -> (128.8323, 126.9871) centre (148.5, 105) ccw
  arc A406 (127.0632, 125.2661) -> (126.5329, 124.69) centre (148.5, 105) ccw
  arc A407 (124.9639, 122.7848) -> (124.5002, 122.154) centre (148.5, 105) ccw
  arc A408 (123.1502, 120.0877) -> (122.7588, 119.4097) centre (148.5, 105) ccw
  arc A409 (121.6443, 117.2075) -> (121.3298, 116.4905) centre (148.5, 105) ccw
  arc A410 (120.4644, 114.179) -> (120.2307, 113.4318) centre (148.5, 105) ccw
  arc A411 (119.6248, 111.0392) -> (119.4747, 110.2708) centre (148.5, 105) ccw
  arc A412 (119.1357, 107.826) -> (119.071, 107.0458) centre (148.5, 105) ccw
  arc A413 (119.003, 104.5785) -> (119.0246, 103.7959) centre (148.5, 105) ccw
  arc A414 (119.2284, 101.3362) -> (119.3359, 100.5607) centre (148.5, 105) ccw
  arc A415 (119.8091, 98.1383) -> (120.0013, 97.3793) centre (148.5, 105) ccw
  arc A416 (120.7381, 95.0237) -> (121.0126, 94.2905) centre (148.5, 105) ccw
  arc A417 (122.0041, 92.0302) -> (122.3576, 91.3317) centre (148.5, 105) ccw
  arc A418 (123.5917, 89.1942) -> (124.0199, 88.5387) centre (148.5, 105) ccw
  arc A419 (125.4816, 86.55) -> (125.9793, 85.9456) centre (148.5, 105) ccw
  arc A420 (127.651, 84.1297) -> (128.2121, 83.5838) centre (148.5, 105) ccw
  arc A421 (130.0734, 81.9628) -> (130.6912, 81.482) centre (148.5, 105) ccw
  arc A422 (132.7195, 80.0756) -> (133.3865, 79.6656) centre (148.5, 105) ccw
  arc A423 (135.5572, 78.4909) -> (136.2652, 78.1567) centre (148.5, 105) ccw
  arc A424 (138.552, 77.228) -> (139.2925, 76.9737) centre (148.5, 105) ccw
  arc A425 (141.6675, 76.3021) -> (142.4315, 76.1309) centre (148.5, 105) ccw
  arc A426 (144.866, 75.7247) -> (145.6441, 75.6386) centre (148.5, 105) ccw
  arc A427 (148.1085, 75.5026) -> (148.8915, 75.5026) centre (148.5, 105) ccw
  arc A428 (151.3559, 75.6386) -> (152.134, 75.7247) centre (148.5, 105) ccw
  arc A429 (154.5685, 76.1309) -> (155.3325, 76.3021) centre (148.5, 105) ccw
  arc A430 (157.7075, 76.9737) -> (158.448, 77.228) centre (148.5, 105) ccw
  arc A431 (160.7348, 78.1567) -> (161.4428, 78.4909) centre (148.5, 105) ccw
  arc A432 (163.6135, 79.6656) -> (164.2805, 80.0756) centre (148.5, 105) ccw
  arc A433 (166.3088, 81.482) -> (166.9266, 81.9628) centre (148.5, 105) ccw
  arc A434 (168.7879, 83.5838) -> (169.349, 84.1297) centre (148.5, 105) ccw
  arc A435 (171.0207, 85.9456) -> (171.5184, 86.55) centre (148.5, 105) ccw
  arc A436 (172.9801, 88.5387) -> (173.4083, 89.1942) centre (148.5, 105) ccw
  arc A437 (174.6424, 91.3317) -> (174.9959, 92.0302) centre (148.5, 105) ccw
  arc A438 (175.9874, 94.2905) -> (176.2619, 95.0237) centre (148.5, 105) ccw
  arc A439 (176.9987, 97.3793) -> (177.1909, 98.1383) centre (148.5, 105) ccw
  arc A440 (177.6641, 100.5607) -> (177.7716, 101.3362) centre (148.5, 105) ccw
  arc A441 (177.9754, 103.7959) -> (177.997, 104.5785) centre (148.5, 105) ccw
  arc A442 (177.929, 107.0458) -> (177.8643, 107.826) centre (148.5, 105) ccw
  arc A443 (177.5253, 110.2708) -> (177.3752, 111.0392) centre (148.5, 105) ccw
  arc A444 (176.7693, 113.4318) -> (176.5356, 114.179) centre (148.5, 105) ccw
  arc A445 (175.6702, 116.4905) -> (175.3557, 117.2075) centre (148.5, 105) ccw
  arc A446 (174.2412, 119.4097) -> (173.8498, 120.0877) centre (148.5, 105) ccw
  arc A447 (172.4998, 122.154) -> (172.0361, 122.7848) centre (148.5, 105) ccw
  arc A448 (170.4671, 124.69) -> (169.9368, 125.2661) centre (148.5, 105) ccw
  arc A449 (168.1677, 126.9871) -> (167.5773, 127.5013) centre (148.5, 105) ccw
  arc A450 (165.6295, 129.0173) -> (164.9862, 129.4634) centre (148.5, 105) ccw
  arc A451 (162.8835, 130.7559) -> (162.1949, 131.1285) centre (148.5, 105) ccw
  arc A452 (159.9628, 132.1819) -> (159.2375, 132.4765) centre (148.5, 105) ccw
  arc A453 (156.903, 133.2779) -> (156.1497, 133.4909) centre (148.5, 105) ccw
  arc A454 (153.7412, 134.0307) -> (152.969, 134.1595) centre (148.5, 105) ccw
  arc A455 (150.5158, 134.431) -> (149.7341, 134.4742) centre (148.5, 105) ccw
  line L0 (117, 105) -> (180, 105)
  line L1 (148.5, 73.5) -> (148.5, 136.5)
  point P0 (0, 0)
  point P1 (149.5, 150)
  point P2 (149.5, 144)
  point P3 (165.6875, 150)
  point P4 (167.8125, 144)
  constraints: 684 point on circle, 342 centre point, 4 end point, 2 horizontal alignment, 344 other
extrude "押し出し1" add sketch "スケッチ1" along normal blind 4